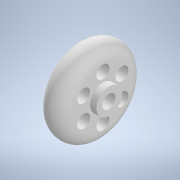
# Autodesk Inventor part: Kolo
Saved by Autodesk Inventor 2022 (Build 260153000, 153)
## iProperties
Created: 2024-01-14
Part Number: Kolo
Material: Generic
Document SubType Name: Modeling
Designer: mateu
Density: 1 g/cm^3
Appearance: Default
Author: mateu
Autodesk Inventor part; units mm, degrees
ref_plane "YZ Plane" through (0, 0, 0) normal (1, 0, 0) x (0, 1, 0)
ref_plane "XZ Plane" through (0, 0, 0) normal (0, 1, 0) x (-1, 0, 0)
ref_plane "XY Plane" through (0, 0, 0) normal (0, 0, 1) x (1, 0, 0)
sketch "Sketch1" plane through (0, 0, 0) normal (0, 0, 1) x (1, 0, 0)
  line L0 (0, 0) -> (30, 0)
  line L1 (30, 0) -> (30, 10)
  line L2 (30, 10) -> (25, 10)
  line L3 (5, 10) -> (0, 10)
  line L4 (0, 10) -> (0, 0)
  line L5 (25, 10) -> (25, 32.1414)
  line L6 (25, 32.1414) -> (5, 32.1414)
  line L7 (5, 32.1414) -> (5, 10)
  constraints: 16 end point, 3 horizontal, 3 perpendicular, 2 point on line, 1 vertical
revolve "Revolution1" add sketch "Sketch1" angle 360 about axis through (0, 0, 0) along (1, 0, 0)
fillet "Fillet1" radius 10 2 edges at (25, -32.1414, 0) (5, -32.1414, 0)
sketch "Sketch2" plane through (30, 0, 0) normal (1, 0, 0) x (0, 0, -1)
  point P0 (0, 0)
  point P1 (-0.0379, -0.3555)
hole "Hole1" at (30, -0.3555, 0.0379) direction (-1, 0, 0) diameter 10 end through all
fillet "Fillet2" radius 0.5 1 edges at (30, -0.3555, 5.0379)
sketch "Sketch3" plane through (25, 0, 0) normal (1, 0, 0) x (0, 0, -1)
  circle A0 centre (-0.0379, -0.3555) radius 5 projected
  circle A1 centre (-0.0379, -0.3555) radius 17.5
  circle A2 centre (0, 17.1445) radius 5
  point P0 (0, 0)
  constraints: 1 centre point, 1 coincident, 3 other
extrude "Extrusion1" cut sketch "Sketch3" along normal through all both and the other way through all contours A2 A1 | A1 A2 picked at (-0.0037, 15.4246) picked at (-0.1177, 18.7538)
pattern_circular "Circular Pattern1" count 6 over 360 about axis through (15, 0, 0) along (1, 0, 0) of "Extrusion1"
body "Solid1"
